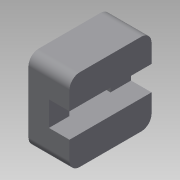
# Autodesk Inventor part: pig_abs
Saved by Autodesk Inventor 2015 (Build 190159000, 159)
## iProperties
Created: 2016-04-29
Part Number: pig_abs
Material: Generic
Document SubType Name: Modeling
Designer: Luke Good
Density: 1 g/cm^3
Appearance: Default
Author: Luke Good
Autodesk Inventor part; units mm, degrees
ref_plane "YZ Plane" through (0, 0, 0) normal (1, 0, 0) x (0, 1, 0)
ref_plane "XZ Plane" through (0, 0, 0) normal (0, 1, 0) x (-1, 0, 0)
ref_plane "XY Plane" through (0, 0, 0) normal (0, 0, 1) x (1, 0, 0)
sketch "Sketch1" plane through (0, 0, 0) normal (0, 0, 1) x (1, 0, 0)
  line L0 (6.35, -12.6955) -> (-6.35, -12.6955)
  line L1 (-6.35, -12.6955) -> (-6.35, 12.6955)
  line L2 (-6.35, 12.6955) -> (6.35, 12.6955)
  line L3 (6.35, 12.6955) -> (6.35, -12.6955)
  line L4 (6.35, -12.6955) -> (-6.35, 12.6955) construction
  line L5 (-6.35, -12.6955) -> (6.35, 12.6955) construction
  point P0 (0, 0)
  dimension "d1" = 0
  dimension "d0" = 12.7
  constraints: 12 end point, 4 point on line, 3 horizontal, 2 midpoint, 2 parallel, 2 vertical, 1 perpendicular, 8 other
  measures "d0" distance of L4.end L2.end
extrude "Extrusion1" add sketch "Sketch1" along normal blind 25.4
fillet "Fillet2" radius 3.175 4 edges at (0, 12.6955, 25.4) (0, -12.6955, 25.4) (0, 12.6955, 0) (0, -12.6955, 0)
sketch "Sketch4" plane through (6.35, -9.5205, 0) normal (1, 0, 0) x (0, 0, -1)
  line L0 (-6.35, 5.0755) -> (-19.05, 13.9655) construction
  line L1 (-19.05, 5.0755) -> (-6.35, 13.9655) construction
  line L2 (-25.4, 0) -> (-25.4, 19.041) projected
  line L3 (-25.4, 13.3305) -> (-25.4, 5.7105)
  line L4 (0, 5.7105) -> (0, 13.3305)
  line L5 (0, 13.9655) -> (-25.4, 5.0755) construction
  line L6 (-25.4, 13.9655) -> (0, 5.0755) construction
  line L7 (0, 5.7105) -> (-25.4, 5.7105)
  line L8 (-25.4, 5.7105) -> (-25.4, 13.3305)
  line L9 (-25.4, 13.3305) -> (0, 13.3305)
  line L10 (0, 13.3305) -> (0, 5.7105)
  line L11 (0, 5.7105) -> (-25.4, 13.3305) construction
  line L12 (-25.4, 5.7105) -> (0, 13.3305) construction
  point P0 (-12.7, 9.5205)
  dimension "d35" = 7.62
  constraints: 24 end point, 6 midpoint, 3 parallel, 1 horizontal, 1 perpendicular, 1 point on line
  measures "d35" distance of L3.start L3.end
extrude "Extrusion4" cut sketch "Sketch4" against normal blind 6.35
sketch "Sketch7" plane through (0, -9.5205, 0) normal (1, 0, 0) x (0, 0, -1)
  line L0 (-6.35, 13.3305) -> (-19.05, 13.3305)
  line L1 (-19.05, 13.3305) -> (-19.05, 5.7105)
  line L2 (-19.05, 5.7105) -> (-6.35, 5.7105)
  line L3 (-6.35, 5.7105) -> (-6.35, 13.3305)
  line L4 (-6.35, 13.3305) -> (-19.05, 5.7105) construction
  line L5 (-19.05, 13.3305) -> (-6.35, 5.7105) construction
  point P0 (0, 9.5205)
  point P1 (-12.7, 9.5205)
  dimension "d36" = 12.7
  dimension "d37" = 7.62
  constraints: 12 end point, 2 midpoint, 2 parallel, 1 horizontal, 1 perpendicular
  measures "d36" distance of L2.end L1.end
  measures "d37" distance of L1.end L0.end
extrude "Extrusion7" cut sketch "Sketch7" against normal blind 12.7
body "Solid1"
